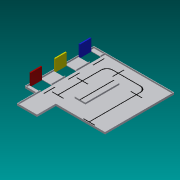
# Autodesk Inventor part: フィールド本体_1
Saved by Autodesk Inventor 2015 (Build 190159000, 159)
## iProperties
Created: 2015-04-21
Part Number: フィールド本体_1
Material: 一般
Document SubType Name: Modeling
Designer: hiroaki
Density: 1 g/cm^3
Appearance: 滑らか - 白
Author: hiroaki
Autodesk Inventor part; units mm, degrees
ref_plane "YZ Plane" through (0, 0, 0) normal (1, 0, 0) x (0, 1, 0)
ref_plane "XZ Plane" through (0, 0, 0) normal (0, 1, 0) x (-1, 0, 0)
ref_plane "XY Plane" through (0, 0, 0) normal (0, 0, 1) x (1, 0, 0)
sketch "スケッチ1" plane through (0, 0, 0) normal (0, 1, 0) x (-1, 0, 0)
  line L0 (-900, 900) -> (900, 900)
  line L1 (900, 900) -> (900, -900)
  line L2 (900, -900) -> (-900, -900)
  line L3 (-900, -900) -> (-900, 900)
  line L4 (-900, 900) -> (900, -900) construction
  line L5 (900, 900) -> (-900, -900) construction
  line L6 (-900, 900) -> (-1400, 900)
  line L7 (-1400, 900) -> (-1400, 400)
  line L8 (-1400, 400) -> (-900, 400)
  line L9 (-900, 400) -> (-900, 900)
  line L10 (900, 900) -> (800, 900)
  line L11 (800, 900) -> (800, 1165)
  line L12 (800, 1165) -> (900, 1165)
  line L13 (900, 1165) -> (900, 900)
  line L14 (500, 900) -> (150, 900)
  line L15 (150, 900) -> (150, 1165)
  line L16 (150, 1165) -> (500, 1165)
  line L17 (500, 1165) -> (500, 900)
  line L18 (650, 900) -> (650, 1196.2048) construction
  line L19 (-150, 900) -> (-500, 900)
  line L20 (-500, 900) -> (-500, 1165)
  line L21 (-500, 1165) -> (-150, 1165)
  line L22 (-150, 1165) -> (-150, 900)
  line L23 (0, 900) -> (0, 1638.8825) construction
  line L24 (-900, 900) -> (-800, 900)
  line L25 (-800, 900) -> (-800, 1165)
  line L26 (-800, 1165) -> (-900, 1165)
  line L27 (-900, 1165) -> (-900, 900)
  line L28 (-650, 900) -> (-650, 1715.6459) construction
  line L29 (-900, 1165) -> (900, 1165)
  line L30 (900, 1165) -> (900, 1195)
  line L31 (900, 1195) -> (-900, 1195)
  line L32 (-900, 1195) -> (-900, 1165)
  point P0 (0, 0)
  dimension "d0" = 1800
  dimension "d1" = 500
  dimension "d2" = 300
  dimension "d3" = 250
  dimension "d4" = 650
  dimension "d5" = 300
  dimension "d7" = 300
  dimension "d9" = 265
  dimension "d10" = 30
  constraints: 66 end point, 15 parallel, 7 horizontal, 7 perpendicular, 6 point on line, 4 equal length, 3 midpoint, 2 vertical, 4 other
  measures "d0" distance of L0.end L1.end
  measures "d1" distance of L6.end L7.end
  measures "d2" distance between parallel lines of L11 L17
  measures "d3" distance between parallel lines of L13 L18
  measures "d4" distance between parallel lines of L18 L23
  measures "d5" distance between parallel lines of L22 L15
  measures "d7" distance between parallel lines of L20 L25
  measures "d9" distance of L12.end L0.end
  measures "d10" distance of L29.end L30.end
extrude "押し出し1" add sketch "スケッチ1" along normal blind 15 contours L27 L26 L25 L0 | L0 L1 L2 L3 | L3 L8 L7 L6 | L32 L31 L30 L12 L29 L16 L21 L26 | L20 L21 L22 L0 | L15 L16 L17 L0 | L0 L11 L12 L13
sketch "スケッチ2" plane through (0, 15, 0) normal (0, 1, 0) x (1, 0, 0)
  line L0 (900, -400) -> (900, 900) projected
  line L1 (900, 900) -> (-900, 900) projected
  line L2 (-900, 900) -> (-900, -1195) projected
  line L3 (-400, -20) -> (500, -20)
  line L4 (500, -20) -> (500, -300)
  line L5 (500, -300) -> (-400, -300)
  line L6 (-400, -300) -> (-400, -20)
  point P0 (0, 0)
  dimension "d13" = 400
  dimension "d14" = 500
  dimension "d15" = 280
  dimension "d16" = 920
  constraints: 8 end point, 2 parallel, 1 horizontal, 1 perpendicular
  measures "d13" distance between parallel lines of L0 L4
  measures "d14" distance between parallel lines of L2 L6
  measures "d15" distance of L5.end L3.start
  measures "d16" distance between parallel lines of L1 L3
extrude "押し出し2" add sketch "スケッチ2" along normal blind 40
sketch "スケッチ4" plane through (0, 0, 0) normal (0, -1, 0) x (1, 0, 0)
  line L0 (900, 900) -> (1400, 900) projected
  line L1 (900, 1195) -> (900, 900) projected
  line L2 (-900, 1195) -> (900, 1195) projected
  line L3 (-900, -900) -> (-900, 1195) projected
  line L4 (900, -900) -> (-900, -900) projected
  line L5 (900, 400) -> (900, -900) projected
  line L6 (1400, 400) -> (900, 400) projected
  line L7 (1400, 900) -> (1400, 400) projected
  line L8 (1412, 388) -> (912, 388)
  line L9 (912, 388) -> (912, -912)
  line L10 (912, -912) -> (-912, -912)
  line L11 (-912, -912) -> (-912, 1207)
  line L12 (-912, 1207) -> (912, 1207)
  line L13 (912, 1207) -> (912, 912)
  line L14 (912, 912) -> (1412, 912)
  line L15 (1412, 912) -> (1412, 388)
  point P0 (0, 0)
  dimension "d19" = 12
  constraints: 16 end point, 7 other
  measures "d19" distance between parallel lines of L14 L0
extrude "押し出し3" add sketch "スケッチ4" against normal blind 55
sketch "スケッチ5" plane through (0, 15, 0) normal (0, 1, 0) x (1, 0, 0)
  line L0 (-500, -1165) -> (-800, -1165) projected
  line L1 (150, -1165) -> (-150, -1165) projected
  line L2 (800, -1165) -> (500, -1165) projected
  line L3 (-900, 900) -> (-900, -1195) projected
  line L4 (-900, -1195) -> (900, -1195) projected
  line L5 (-800, -900) -> (-900, -900)
  line L6 (-800, -900) -> (-500, -900) projected
  line L7 (-500, -900) -> (-150, -900)
  line L8 (150, -900) -> (500, -900)
  line L9 (-150, -900) -> (150, -900) projected
  line L10 (800, -900) -> (900, -900)
  line L11 (-800, -1165) -> (-800, -1195)
  line L12 (-500, -1165) -> (-500, -1195)
  line L13 (150, -1165) -> (150, -1195)
  line L14 (-150, -1165) -> (-150, -1195)
  line L15 (500, -1165) -> (500, -1195)
  line L16 (800, -1165) -> (800, -1195)
  point P0 (0, 0)
  constraints: 20 end point, 7 point on line, 4 collinear, 4 perpendicular, 1 parallel, 1 vertical
extrude "押し出し4" add sketch "スケッチ5" along normal blind 300
sketch "スケッチ6" plane through (0, 15, 0) normal (0, 1, 0) x (1, 0, 0)
  line L0 (-150, -1165) -> (-150, -900) projected
  line L1 (150, -900) -> (150, -1165) projected
  line L2 (900, -1195) -> (900, -900) projected
  line L3 (-900, 900) -> (-900, -1195) projected
  line L4 (-800, -900) -> (-900, -900)
  line L5 (-900, -900) -> (-900, -912)
  line L6 (-900, -912) -> (-800, -912)
  line L7 (-800, -912) -> (-800, -900)
  line L8 (-500, -900) -> (-150, -900)
  line L9 (-150, -900) -> (-150, -912)
  line L10 (-150, -912) -> (-500, -912)
  line L11 (-500, -912) -> (-500, -900)
  line L12 (500, -900) -> (150, -900)
  line L13 (150, -900) -> (150, -912)
  line L14 (150, -912) -> (500, -912)
  line L15 (500, -912) -> (500, -900)
  line L16 (800, -900) -> (900, -900)
  line L17 (900, -900) -> (900, -912)
  line L18 (900, -912) -> (800, -912)
  line L19 (800, -912) -> (800, -900)
  point P0 (0, 0)
  dimension "d24" = 12
  constraints: 32 end point, 8 parallel, 5 point on line, 4 horizontal, 4 perpendicular, 3 horizontal alignment
  measures "d24" distance between parallel lines of L4 L6
extrude "押し出し5" add sketch "スケッチ6" along normal blind 40
sketch "スケッチ7" plane through (0, 15, 0) normal (0, 1, 0) x (1, 0, 0)
  line L0 (900, -400) -> (900, 900) projected
  line L1 (900, 900) -> (-900, 900) projected
  line L2 (-900, 900) -> (-900, -900) projected
  line L3 (-800, -900) -> (-500, -900) projected
  line L4 (-500, -900) -> (-150, -900) projected
  line L5 (500, -830) -> (800, -830)
  line L6 (800, -830) -> (800, -810)
  line L7 (800, -810) -> (500, -810)
  line L8 (500, -810) -> (500, -830)
  line L9 (-150, -830) -> (150, -830)
  line L10 (150, -830) -> (150, -810)
  line L11 (150, -810) -> (-150, -810)
  line L12 (-150, -810) -> (-150, -830)
  line L13 (-800, -830) -> (-500, -830)
  line L14 (-500, -830) -> (-500, -810)
  line L15 (-500, -810) -> (-800, -810)
  line L16 (-800, -810) -> (-800, -830)
  line L17 (660, -750) -> (660, -450)
  line L18 (660, -450) -> (640, -450)
  line L19 (640, -450) -> (640, -590)
  line L20 (640, -590) -> (10, -590)
  line L21 (10, -590) -> (10, -450)
  line L22 (10, -450) -> (-10, -450)
  line L23 (-10, -450) -> (-10, -590)
  line L24 (-10, -590) -> (-490, -590)
  line L25 (-640, -440) -> (-640, -310)
  line L26 (-640, -310) -> (-500, -310)
  line L27 (-500, -310) -> (-500, -290)
  line L28 (-500, -290) -> (-640, -290)
  line L29 (-640, -290) -> (-640, 270)
  arc A0 (-490, 420) -> (-640, 270) centre (-490, 270) ccw
  line L30 (-490, 420) -> (-410, 420)
  line L31 (-410, 420) -> (-410, 280)
  line L32 (-410, 280) -> (-390, 280)
  line L33 (-390, 280) -> (-390, 420)
  line L34 (-390, 420) -> (840, 420)
  line L35 (840, 420) -> (840, 280)
  line L36 (840, 280) -> (860, 280)
  line L37 (860, 280) -> (860, 420)
  line L38 (860, 420) -> (900, 420)
  arc A1 (-640, -440) -> (-490, -590) centre (-490, -440) ccw
  line L39 (0, -450) -> (0, -597.588) construction
  line L40 (650, -450) -> (650, -650) construction
  line L41 (850, 280) -> (850, 559.6959) construction
  line L42 (-400, 280) -> (-400, 450.6636) construction
  line L43 (660, -750) -> (640, -750)
  line L44 (640, -750) -> (640, -610)
  line L45 (640, -610) -> (10, -610)
  line L46 (10, -610) -> (10, -750)
  line L47 (10, -750) -> (-10, -750)
  line L48 (-10, -750) -> (-10, -610)
  line L49 (-10, -610) -> (-510, -610)
  line L50 (0, -600) -> (-123.7185, -600) construction
  arc A2 (-660, -460) -> (-510, -610) centre (-510, -460) ccw
  line L51 (-660, -460) -> (-660, -310)
  line L52 (-660, -310) -> (-800, -310)
  line L53 (-800, -310) -> (-800, -290)
  line L54 (-800, -290) -> (-660, -290)
  line L55 (-660, -290) -> (-660, 290)
  line L56 (-800, -300) -> (-500, -300) construction
  line L57 (-650, -300) -> (-650, -220.6118) construction
  arc A3 (-510, 440) -> (-660, 290) centre (-510, 290) ccw
  line L58 (-510, 440) -> (-410, 440)
  line L59 (-410, 440) -> (-410, 580)
  line L60 (-410, 580) -> (-390, 580)
  line L61 (-390, 580) -> (-390, 440)
  line L62 (-390, 440) -> (840, 440)
  line L63 (840, 440) -> (840, 580)
  line L64 (840, 580) -> (860, 580)
  line L65 (860, 580) -> (860, 440)
  line L66 (860, 440) -> (900, 440)
  point P0 (500, -900)
  point P1 (0, 0)
  point P2 (850, 580)
  point P3 (-400, 580)
  dimension "d27" = 300
  dimension "d28" = 20
  dimension "d29" = 70
  dimension "d30" = 150
  dimension "d32" = 150
  dimension "d33" = 20
  dimension "d34" = 300
  dimension "d35" = 480
  dimension "d36" = 650
  dimension "d37" = 250
  dimension "d38" = 50
  dimension "d39" = 500
  dimension "d40" = 20
  dimension "d41" = 300
  dimension "d42" = 20
  dimension "d43" = 300
  dimension "d44" = 250
  dimension "d45" = 20
  constraints: 124 end point, 33 perpendicular, 19 equal length, 11 vertical, 10 vertical alignment, 9 horizontal alignment, 9 midpoint, 8 horizontal, 8 parallel, 8 point on circle, 8 tangent, 7 point on line, 4 centre point, 2 equal radius, 1 other
  measures "d27" distance of L10.end L11.end
  measures "d28" distance of L11.end L9.start
  measures "d29" distance between parallel lines of L3 L13
  measures "d30" radius of A1
  measures "d32" radius of A0
  measures "d33" distance of L17.end L18.end
  measures "d34" distance of L17.start L17.end
  measures "d35" distance between parallel lines of L1 L30
  measures "d36" distance between parallel lines of L39 L40
  measures "d37" distance between parallel lines of L0 L40
  measures "d38" distance between parallel lines of L0 L41
  measures "d39" distance between parallel lines of L2 L42
  measures "d40" distance between parallel lines of L24 L49
  measures "d41" distance between parallel lines of L4 L50
  measures "d42" distance between parallel lines of L51 L25
  measures "d43" distance between parallel lines of L50 L56
  measures "d44" distance between parallel lines of L2 L57
  measures "d45" distance between parallel lines of L62 L34
extrude "押し出し6" add sketch "スケッチ7" along normal blind 0.001
sketch "スケッチ8" plane through (0, 55, 0) normal (0, 1, 0) x (1, 0, 0)
  line L0 (-400, -300) -> (500, -300) projected
  line L1 (500, -300) -> (500, -20) projected
  line L2 (-400, -300) -> (-400, -20) projected
  line L3 (-400, -170) -> (500, -170)
  line L4 (500, -170) -> (500, -150)
  line L5 (500, -150) -> (-400, -150)
  line L6 (-400, -150) -> (-400, -170)
  line L7 (-327.3168, -160) -> (-261.4952, -160) construction
  point P0 (0, 0)
  dimension "d48" = 20
  dimension "d49" = 140
  constraints: 10 end point, 2 horizontal, 2 parallel, 2 point on line, 1 perpendicular, 1 other
  measures "d48" distance between parallel lines of L5 L3
  measures "d49" distance between parallel lines of L0 L7
extrude "押し出し7" add sketch "スケッチ8" along normal blind 0.001 contours L2 L5 L1 L3
equation "\"d5\" = d2"
equation "\"d7\" = d5"
equation "\"d28\" = 線の太さ"
equation "\"d32\" = d30"
equation "\"d33\" = 線の太さ"
equation "\"d40\" = 線の太さ"
equation "\"d42\" = 線の太さ"
equation "\"d43\" = d41"
equation "\"d45\" = 線の太さ"
equation "\"d48\" = 線の太さ"
equation "\"d50\" = d46"
equation "\"線の太さ\" = 20"
equation "\"d46\" = 0.001"
